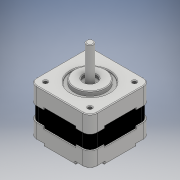
# Autodesk Inventor part: NEMA-17_17HS4401
Saved by Autodesk Inventor 2018 (Build 220112000, 112)
## iProperties
Created: 2018-09-20
Part Number: NEMA-17_17HS4401
Material: Genérico
Document SubType Name: Modeling
Designer: Georgines
Density: 1 g/cm^3
Appearance: Padrão
Author: Georgines
Autodesk Inventor part; units mm, degrees
ref_plane "YZ Plane" through (0, 0, 0) normal (1, 0, 0) x (0, 1, 0)
ref_plane "XZ Plane" through (0, 0, 0) normal (0, 1, 0) x (-1, 0, 0)
ref_plane "XY Plane" through (0, 0, 0) normal (0, 0, 1) x (1, 0, 0)
sketch "Esboço1" plane through (0, 0, 0) normal (0, 0, 1) x (1, 0, 0)
  line L0 (-16.15, -21.15) -> (16.15, -21.15)
  line L1 (21.15, -16.15) -> (21.15, 16.15)
  line L2 (16.15, 21.15) -> (-16.15, 21.15)
  line L3 (-21.15, 16.15) -> (-21.15, -16.15)
  line L4 (-21.15, -21.15) -> (21.15, 21.15) construction
  line L5 (21.15, -21.15) -> (-21.15, 21.15) construction
  arc A0 (16.15, -21.15) -> (21.15, -16.15) centre (16.15, -16.15) ccw
  arc A1 (21.15, 16.15) -> (16.15, 21.15) centre (16.15, 16.15) ccw
  arc A2 (-16.15, 21.15) -> (-21.15, 16.15) centre (-16.15, 16.15) ccw
  arc A3 (-21.15, -16.15) -> (-16.15, -21.15) centre (-16.15, -16.15) ccw
  point P0 (0, 0)
  dimension "d0" = 42.3
  dimension "d1" = 42.3
  dimension "d67" = 5
  constraints: 12 end point, 8 point on circle, 8 point on line, 8 tangent, 4 centre point, 3 equal radius, 2 midpoint, 2 parallel, 1 horizontal, 1 perpendicular
  measures "d0" distance of L4.end L5.end
  measures "d1" distance of L5.start L4.end
  measures "d67" radius of A0
extrude "Extrusão1" add sketch "Esboço1" along normal blind 12
sketch "Esboço2" plane through (0, 0, 0) normal (0, 0, -1) x (-1, 0, 0)
  line L0 (21.15, 16.15) -> (21.15, -16.15) projected
  circle A0 centre (21.15, 21.15) radius 10
  line L1 (-21.15, -16.15) -> (-21.15, 16.15) projected
  circle A1 centre (-21.15, 21.15) radius 10
  circle A2 centre (-21.15, -21.15) radius 10
  circle A3 centre (21.15, -21.15) radius 10
  line L2 (21.15, 0) -> (-21.15, 0) construction
  line L3 (0, -21.2295) -> (0, 21.15) construction
  line L4 (-16.15, 21.15) -> (16.15, 21.15) construction
  point P0 (0, 0)
  dimension "d5" = 20
  dimension "d6" = 20
  dimension "d7" = 20
  dimension "d8" = 20
  dimension "d68" = 21.15
  dimension "d69" = 21.15
  dimension "d70" = 21.15
  dimension "d71" = 21.15
  dimension "d72" = 21.15
  dimension "d73" = 21.15
  dimension "d74" = 21.15
  dimension "d75" = 21.15
  constraints: 4 centre point, 4 end point, 3 midpoint, 2 coincident
  measures "d5" diameter of A0
  measures "d6" diameter of A1
  measures "d7" diameter of A2
  measures "d8" diameter of A3
  measures "d68" distance from line of L2 point (21.15, -21.15)
  measures "d69" distance from line of L3 point (21.15, -21.15)
  measures "d70" distance from line of L3 point (-21.15, -21.15)
  measures "d71" distance from line of L2 point (-21.15, -21.15)
  measures "d72" distance from line of A0.centre L3
  measures "d73" distance from line of A0.centre L2
  measures "d74" distance from line of L2 A1.centre
  measures "d75" distance from line of L3 A1.centre
extrude "Extrusão2" cut sketch "Esboço2" against normal blind 1.5
sketch "Esboço3" plane through (0, 0, 0) normal (0, 0, -1) x (-1, 0, 0)
  circle A0 centre (0, 0) radius 4.5
  dimension "d11" = 9
  constraints: 1 centre point, 1 coincident
  measures "d11" diameter of A0
extrude "Extrusão3" cut sketch "Esboço3" against normal blind 1.5
sketch "Esboço5" plane through (0, 0, 12) normal (0, 0, 1) x (1, 0, 0)
  line L0 (-11.15, 21.15) -> (11.182, 21.15)
  line L1 (11.182, -21.2685) -> (-11.15, -21.2685)
  line L2 (-21.15, 11.15) -> (-21.15, -11.15) projected
  line L3 (-21.15, 11.15) -> (-21.15, -11.15)
  line L4 (21.15, -11.15) -> (21.15, 11.15)
  line L5 (-11.15, -21.2685) -> (-11.15, -20.5)
  line L6 (-11.15, 20.5) -> (-11.15, 21.15)
  line L7 (21.15, 11.15) -> (20.5, 11.15)
  line L8 (-20.5, 11.15) -> (-21.15, 11.15)
  line L9 (-21.15, -11.15) -> (-20.5, -11.15)
  line L10 (20.5, -11.15) -> (21.15, -11.15)
  line L11 (-20.5, 20.5) -> (20.5, -20.5) construction
  line L12 (20.5, 20.5) -> (-20.5, -20.5) construction
  line L13 (-20.5, -15.5) -> (-20.5, -11.15)
  line L14 (-20.5, 11.15) -> (-20.5, 15.5)
  line L15 (11.182, 21.15) -> (11.182, 20.3504)
  line L16 (11.182, 11.182) -> (11.182, 11.15)
  line L17 (20.5, 15.5) -> (20.5, 11.15)
  line L18 (20.5, -11.15) -> (20.5, -15.5)
  line L19 (11.182, -11.15) -> (11.182, -11.182)
  line L20 (11.182, -20.5) -> (11.182, -21.2685)
  line L21 (15.5, -20.5) -> (11.182, -20.5)
  line L22 (-11.15, -20.5) -> (-15.5, -20.5)
  line L23 (-15.5, 20.5) -> (-11.15, 20.5)
  line L24 (11.182, 20.5) -> (15.5, 20.5)
  arc A0 (-20.5, -15.5) -> (-15.5, -20.5) centre (-15.5, -15.5) ccw
  arc A1 (15.5, -20.5) -> (20.5, -15.5) centre (15.5, -15.5) ccw
  arc A2 (20.5, 15.5) -> (15.5, 20.5) centre (15.5, 15.5) ccw
  arc A3 (-15.5, 20.5) -> (-20.5, 15.5) centre (-15.5, 15.5) ccw
  point P0 (0, 0)
  dimension "d16" = 41
  dimension "d17" = 41
  dimension "d66" = 5
  constraints: 48 end point, 22 parallel, 11 point on line, 10 perpendicular, 8 point on circle, 8 tangent, 5 horizontal, 4 centre point, 3 equal radius, 2 midpoint
  measures "d16" distance of L11.end L12.end
  measures "d17" distance of L12.start L11.end
  measures "d66" radius of A0
extrude "Extrusão4" cut sketch "Esboço5" against normal blind 1.5
sketch "Esboço6" plane through (0, 0, 10.5) normal (0, 0, 1) x (1, 0, 0)
  line L0 (-15.5, -20.5) -> (15.5, -20.5)
  line L1 (20.5, -15.5) -> (20.5, 15.5)
  line L2 (15.5, 20.5) -> (-15.5, 20.5)
  line L3 (-20.5, 15.5) -> (-20.5, -15.5)
  line L4 (-20.5, -20.5) -> (20.5, 20.5) construction
  line L5 (20.5, -20.5) -> (-20.5, 20.5) construction
  arc A0 (20.5, 15.5) -> (15.5, 20.5) centre (15.5, 15.5) ccw
  arc A1 (15.5, -20.5) -> (20.5, -15.5) centre (15.5, -15.5) ccw
  arc A2 (-20.5, -15.5) -> (-15.5, -20.5) centre (-15.5, -15.5) ccw
  arc A3 (-15.5, 20.5) -> (-20.5, 15.5) centre (-15.5, 15.5) ccw
  point P0 (0, 0)
  dimension "d20" = 41
  dimension "d21" = 41
  dimension "d65" = 5
  constraints: 12 end point, 8 point on circle, 8 point on line, 8 tangent, 4 centre point, 3 equal radius, 2 midpoint, 2 parallel, 1 horizontal, 1 perpendicular
  measures "d20" distance of L5.end L4.end
  measures "d21" distance of L4.end L5.start
  measures "d65" radius of A0
extrude "Extrusão5" add sketch "Esboço6" along normal blind 13
sketch "Esboço8" plane through (0, 0, 23.5) normal (0, 0, 1) x (1, 0, 0)
  line L0 (16.15, -21.15) -> (-16.15, -21.15)
  line L1 (-21.15, -16.15) -> (-21.15, 16.15)
  line L2 (-16.15, 21.15) -> (16.15, 21.15)
  line L3 (21.15, 16.15) -> (21.15, -16.15)
  line L4 (21.15, -21.15) -> (-21.15, 21.15) construction
  line L5 (-21.15, -21.15) -> (21.15, 21.15) construction
  line L6 (-11.15, 21.15) -> (11.182, 21.15)
  line L7 (-21.15, 11.15) -> (-21.15, -11.15)
  line L8 (-21.15, 11.15) -> (-21.15, -11.15)
  line L9 (21.15, -11.15) -> (21.15, 11.15)
  line L10 (-11.15, 20.5) -> (-11.15, 21.15)
  line L11 (21.15, 11.15) -> (20.5, 11.15)
  line L12 (-20.5, 11.15) -> (-21.15, 11.15)
  line L13 (-21.15, -11.15) -> (-20.5, -11.15)
  line L14 (20.5, -11.15) -> (21.15, -11.15)
  line L15 (-20.5, 20.5) -> (20.5, -20.5) construction
  line L16 (20.5, 20.5) -> (-20.5, -20.5) construction
  line L17 (-20.5, -15.5) -> (-20.5, -11.15)
  line L18 (-20.5, 11.15) -> (-20.5, 15.5)
  line L19 (11.182, 21.15) -> (11.182, 20.3504)
  line L20 (11.182, 11.182) -> (11.182, 11.15)
  line L21 (20.5, 15.5) -> (20.5, 11.15)
  line L22 (20.5, -11.15) -> (20.5, -15.5)
  line L23 (11.182, -11.15) -> (11.182, -11.182)
  line L24 (15.5, -20.5) -> (11.182, -20.5)
  line L25 (-11.15, -20.5) -> (-15.5, -20.5)
  line L26 (-15.5, 20.5) -> (-11.15, 20.5)
  line L27 (11.182, 20.5) -> (15.5, 20.5)
  line L28 (11.182, -20.5) -> (11.182, -21.15)
  line L29 (-11.15, -21.15) -> (11.15, -21.15)
  line L30 (-11.15, -21.15) -> (-11.15, -20.5)
  line L31 (-11.15, -21.15) -> (11.182, -21.15)
  arc A0 (21.15, 16.15) -> (16.15, 21.15) centre (16.15, 16.15) ccw
  arc A1 (20.5, 15.5) -> (15.5, 20.5) centre (15.5, 15.5) ccw
  arc A2 (16.15, -21.15) -> (21.15, -16.15) centre (16.15, -16.15) ccw
  arc A3 (15.5, -20.5) -> (20.5, -15.5) centre (15.5, -15.5) ccw
  arc A4 (-20.5, -15.5) -> (-15.5, -20.5) centre (-15.5, -15.5) ccw
  arc A5 (-21.15, -16.15) -> (-16.15, -21.15) centre (-16.15, -16.15) ccw
  arc A6 (-16.15, 21.15) -> (-21.15, 16.15) centre (-16.15, 16.15) ccw
  arc A7 (-15.5, 20.5) -> (-20.5, 15.5) centre (-15.5, 15.5) ccw
  point P0 (0, 0)
  point P1 (0, 0)
  dimension "d26" = 41
  dimension "d27" = 41
  dimension "d64" = 5
  constraints: 64 end point, 20 point on line, 16 point on circle, 8 centre point, 4 midpoint
  measures "d26" distance of L15.end L16.end
  measures "d27" distance of L16.start L15.end
  measures "d64" radius of A0
extrude "Extrusão6" add sketch "Esboço8" against normal blind 1.5 contours L0 L28 L24 A3 L22 L14 L3 A2 | L0 A5 L1 L13 L17 A4 L25 L30 | L11 L21 A1 L27 L19 L2 A0 L3 | L1 A6 L2 L10 L26 A7 L18 L12
sketch "Esboço9" plane through (0, 0, 23.5) normal (0, 0, 1) x (1, 0, 0)
  line L0 (11.182, 21.15) -> (-11.15, 21.15)
  line L1 (-16.15, -21.15) -> (16.15, -21.15)
  line L2 (21.15, -16.15) -> (21.15, 16.15)
  line L3 (16.15, 21.15) -> (-16.15, 21.15)
  line L4 (-21.15, 16.15) -> (-21.15, -16.15)
  line L5 (-21.15, -21.15) -> (21.15, 21.15) construction
  line L6 (21.15, -21.15) -> (-21.15, 21.15) construction
  arc A0 (21.15, 16.15) -> (16.15, 21.15) centre (16.15, 16.15) ccw
  arc A1 (16.15, -21.15) -> (21.15, -16.15) centre (16.15, -16.15) ccw
  arc A2 (-21.15, -16.15) -> (-16.15, -21.15) centre (-16.15, -16.15) ccw
  arc A3 (-16.15, 21.15) -> (-21.15, 16.15) centre (-16.15, 16.15) ccw
  point P0 (0, 0)
  dimension "d62" = 5
  dimension "d63" = 5
  constraints: 14 end point, 8 point on circle, 8 point on line, 4 centre point, 2 midpoint
  measures "d62" radius of A0
  measures "d63" radius of A1
extrude "Extrusão7" add sketch "Esboço9" along normal blind 10.5
sketch "Esboço10" plane through (0, 0, 34) normal (0, 0, 1) x (1, 0, 0)
  circle A0 centre (0, 0) radius 11
  circle A1 centre (0, 0) radius 13.3093
  dimension "d32" = 22
  constraints: 2 centre point, 2 coincident
  measures "d32" diameter of A0
extrude "Extrusão8" cut sketch "Esboço10" against normal blind 1
sketch "Esboço11" plane through (0, 0, 34) normal (0, 0, 1) x (1, 0, 0)
  circle A0 centre (0, 0) radius 11
  dimension "d35" = 22
  constraints: 1 centre point, 1 coincident
  measures "d35" diameter of A0
extrude "Extrusão9" add sketch "Esboço11" along normal blind 2
sketch "Esboço12" plane through (0, 0, 36) normal (0, 0, 1) x (1, 0, 0)
  circle A0 centre (0, 0) radius 4.5
  constraints: 1 centre point, 1 coincident
extrude "Extrusão10" cut sketch "Esboço12" against normal blind 2
sketch "Esboço13" plane through (0, 0, 34) normal (0, 0, 1) x (1, 0, 0)
  circle A0 centre (0, 0) radius 2.5
  dimension "d40" = 5
  constraints: 1 centre point, 1 coincident
  measures "d40" diameter of A0
extrude "Extrusão11" add sketch "Esboço13" along normal blind 24
sketch "Esboço14" plane through (0, 0, 34) normal (0, 0, 1) x (1, 0, 0)
  circle A0 centre (15.5, -15.5369) radius 1
  circle A1 centre (-15.5, -15.5057) radius 1
  circle A2 centre (-15.5, 15.4943) radius 1
  circle A3 centre (15.5, 15.4631) radius 1
  line L0 (-16.15, -21.15) -> (16.15, -21.15) construction
  line L1 (0, -21.15) -> (0, 21.1439) construction
  line L2 (21.2721, -0.0427) -> (-21.15, 0) construction
  line L3 (-21.15, 16.15) -> (-21.15, -16.15) construction
  point P0 (0, 0)
  point P1 (-21.15, -21.15)
  point P2 (21.15, -21.15)
  point P3 (-21.15, 21.15)
  dimension "d43" = 15.5
  dimension "d44" = 15.5
  dimension "d45" = 15.5
  dimension "d46" = 15.5
  dimension "d47" = 15.5
  dimension "d48" = 15.5
  dimension "d49" = 15.5
  dimension "d50" = 15.5
  dimension "d51" = 2
  dimension "d52" = 2
  dimension "d53" = 2
  dimension "d54" = 2
  constraints: 4 centre point, 4 end point, 2 midpoint, 1 vertical
  measures "d43" distance from line of L2 A1.centre
  measures "d44" distance from line of A1.centre L1
  measures "d45" distance from line of L1 A0.centre
  measures "d46" distance from line of L1 A3.centre
  measures "d47" distance from line of L1 A2.centre
  measures "d48" distance from line of L2 A2.centre
  measures "d49" distance from line of L2 A3.centre
  measures "d50" distance from line of L2 A0.centre
  measures "d51" diameter of A0
  measures "d52" diameter of A1
  measures "d53" diameter of A2
  measures "d54" diameter of A3
hole "Furo1" at (-15.5, -15.5057, 34) at (15.5, 15.4631, 34) at (15.5, -15.5369, 34) at (-15.5, 15.4943, 34) direction (0, 0, -1) diameter 2.459 end through all thread size "M3x0.5" class "6H" standard "ANSI Metric M Profile"
fillet "Arredondamento2" radius 0.5 2 edges at (-11, 0, 36) (-4.5, 0, 36)
fillet "Arredondamento3" radius 0.5 17 edges at (-19.6855, -19.6855, 1.5) (-13.65, -21.15, 1.5) (-21.15, -13.65, 1.5) (-21.15, 13.65, 1.5) (-13.65, 21.15, 1.5) (-19.6855, 19.6855, 1.5) (13.65, 21.15, 1.5) (21.15, 13.65, 1.5) (19.6855, 19.6855, 1.5) (19.6855, -19.6855, 1.5) (13.65, -21.15, 1.5) (21.15, -13.65, 1.5) (-14.0789, 14.0789, 0) (14.0789, 14.0789, 0) (14.0789, -14.0789, 0) (-14.0789, -14.0789, 0) (4.5, 0, 0)
fillet "Arredondamento4" radius 0.5 28 edges at (-11.0036, 21.15, 0.1464) (-11.15, 21.15, 1) (-11.15, 21.15, 1.75) (11.0036, 21.15, 0.1464) (11.15, 21.15, 1) (11.15, 21.15, 1.75) (0, 21.15, 0) (11.0036, -21.15, 0.1464) (11.15, -21.15, 1) (11.15, -21.15, 1.75) (-11.0036, -21.15, 0.1464) (-11.15, -21.15, 1) (-11.15, -21.15, 1.75) (0, -21.15, 0) (-21.15, -11.0036, 0.1464) (-21.15, -11.15, 1) (-21.15, -11.15, 1.75) (-21.15, 11.0036, 0.1464) (-21.15, 11.15, 1) (-21.15, 11.15, 1.75) (-21.15, 0, 0) (21.15, 11.0036, 0.1464) (21.15, 11.15, 1) (21.15, 11.15, 1.75) (21.15, -11.0036, 0.1464) (21.15, -11.15, 1) (21.15, -11.15, 1.75) (21.15, 0, 0)
fillet "Arredondamento5" radius 0.5 9 edges at (0, -21.15, 34) (19.6855, -19.6855, 34) (21.15, 0, 34) (19.6855, 19.6855, 34) (0, 21.15, 34) (-19.6855, 19.6855, 34) (-21.15, 0, 34) (-19.6855, -19.6855, 34) (-13.3093, 0, 34)
fillet "Arredondamento6" radius 0.5 8 edges at (-15.5, 16.7238, 34) (15.5, 16.6926, 34) (15.5, -14.3074, 34) (-15.5, -14.2762, 34) (-15.5, 16.7238, 1.5) (-15.5, -14.2762, 1.5) (15.5, 16.6926, 1.5) (15.5, -14.3074, 1.5)
sketch "Esboço15" plane through (0, 0, 1.5) normal (0, 0, -1) x (-1, 0, 0)
  circle A0 centre (0, 0) radius 2.5 projected
  circle A1 centre (0, 0) radius 2.5
  dimension "d81" = 5
  constraints: 1 centre point, 1 coincident
  measures "d81" diameter of A1
extrude "Extrusão12" add sketch "Esboço15" along normal blind 1.5
fillet "Arredondamento7" radius 0.5 1 edges at (2.5, 0, 0)
fillet "Arredondamento8" radius 0.5 1 edges at (-2.5, 0, 58)
equation "\"d1\" = d0"
equation "\"d6\" = d5"
equation "\"d7\" = d5"
equation "\"d8\" = d5"
equation "\"d45\" = d44"
equation "\"d46\" = d44"
equation "\"d47\" = d44"
equation "\"d48\" = d43"
equation "\"d49\" = d43"
equation "\"d50\" = d43"
equation "\"d52\" = d51"
equation "\"d53\" = d51"
equation "\"d54\" = d51"
